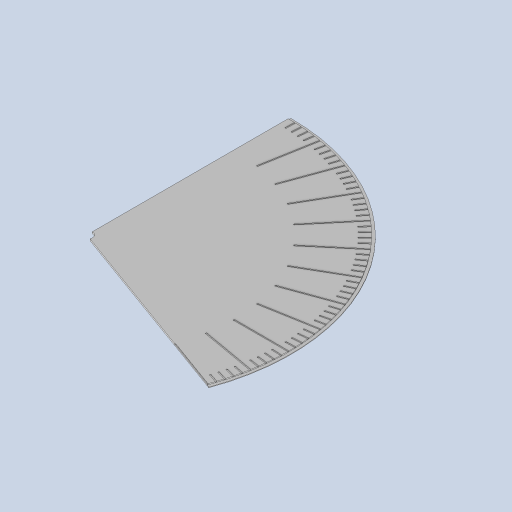
# Autodesk Inventor part: back_angler
Saved by Autodesk Inventor 2024.1 (Build 281209000, 209)
## iProperties
Created: 2023-12-04
Part Number: back_angler
Material: Generic
Document SubType Name: Modeling
Designer: dsdan
Density: 1 g/cm^3
Appearance: Default
Author: dsdan
Autodesk Inventor part; units mm, degrees
ref_plane "YZ Plane" through (0, 0, 0) normal (1, 0, 0) x (0, 1, 0)
ref_plane "XZ Plane" through (0, 0, 0) normal (0, 1, 0) x (-1, 0, 0)
ref_plane "XY Plane" through (0, 0, 0) normal (0, 0, 1) x (1, 0, 0)
sketch "Sketch1" plane through (0, 0, 0) normal (0, 1, 0) x (-1, 0, 0)
  circle A0 centre (0, 0) radius 111.8
  line L0 (0, 111.8) -> (0, -111.8)
  dimension "d0" = 223.6
  constraints: 2 end point, 2 point on circle, 1 centre point, 1 coincident, 1 vertical
  measures "d0" diameter of A0
extrude "Extrusion1" add sketch "Sketch1" along normal blind 0.6 contours L0 A0 picked at (-22.6865, 29.5656)
sketch "Sketch2" plane through (0, 0.6, 0) normal (0, 1, 0) x (1, 0, 0)
  arc A0 (0, -111.8) -> (0, 111.8) centre (0, 0) ccw projected
  line L0 (0, 111.8) -> (0, -111.8) projected
  line L1 (3.9018, -111.7319) -> (3.7272, -106.7319)
  line L2 (19.7832, -110.0364) -> (14.5737, -80.4922)
  line L3 (13.8351, -80.6224) -> (19.0446, -110.1666)
  arc A1 (19.0446, -110.1666) -> (19.7832, -110.0364) centre (19.4139, -110.1015) ccw
  arc A2 (14.5737, -80.4922) -> (13.8351, -80.6224) centre (14.2044, -80.5573) ccw
  line L4 (3.7272, -106.7319) -> (3.9018, -111.7319) construction
  line L5 (3.3524, -106.745) -> (3.527, -111.745)
  line L6 (4.2765, -111.7188) -> (4.1019, -106.7188)
  arc A3 (4.1019, -106.7188) -> (3.3524, -106.745) centre (3.7272, -106.7319) ccw
  arc A4 (3.527, -111.745) -> (4.2765, -111.7188) centre (3.9018, -111.7319) ccw
  line L7 (19.4139, -110.1015) -> (14.2044, -80.5573)
  point P0 (3.8145, -109.2319)
  point P1 (3.527, -111.7444)
  point P2 (4.2765, -111.7182)
  dimension "d9" = 5
  dimension "d14" = 0.75
  dimension "d15" = 0.75
  dimension "d26" = 2
  dimension "d27" = 30
  dimension "d28" = 10
  constraints: 16 end point, 10 point on circle, 8 tangent, 4 centre point, 3 midpoint, 2 parallel, 2 point on line
  measures "d9" vertical distance of L1.start L1.end
  measures "d14" diameter of A2
  measures "d15" diameter of A4
  measures "d26" angle of L0 L1
  measures "d27" distance of L7.start L7.end
  measures "d28" angle of L0 L7
extrude "Extrusion2" cut sketch "Sketch2" against normal blind 0.3 contours A0 A4 | A1 A0 | A0 L3 A2 L2
extrude "Extrusion3" cut sketch "Sketch2" against normal blind 0.3 contours L5 A3 L6 A0
pattern_circular "Circular Pattern1" count 89 over 176 about axis through (0, -10, 0) along (0, 1, 0) of "Extrusion3"
pattern_circular "Circular Pattern2" count 17 over 160 about axis through (0, -10, 0) along (0, 1, 0) of "Extrusion2"
sketch "Sketch3" plane through (0, 0.6, 0) normal (0, 1, 0) x (1, 0, 0)
  circle A0 centre (0, 0) radius 3
  dimension "d29" = 6
  constraints: 1 centre point, 1 coincident
  measures "d29" diameter of A0
extrude "Extrusion4" cut sketch "Sketch3" against normal through all
sketch "Sketch4" plane through (0, 0, 0) normal (0, -1, 0) x (1, 0, 0)
  arc A0 (0, -3) -> (0, 3) centre (0, 0) ccw projected
  line L0 (0, -111.8) -> (0, -3) projected
  arc A1 (0, -111.8) -> (0, 111.8) centre (0, 0) ccw projected
  line L1 (0, 3) -> (0, 111.8) projected
  arc A2 (-1.5, -113.2901) -> (-1.5, 113.2901) centre (0, 0) ccw
  line L2 (0, -111.8) -> (0, -113.3)
  line L3 (0, 111.8) -> (0, 113.3)
  dimension "d32" = 1.5
  constraints: 4 end point, 4 point on circle, 1 centre point, 1 point on line, 1 vertical
  measures "d32" radial gap between concentric circles of A1 A2
extrude "Extrusion5" add sketch "Sketch4" along normal blind 0.3
sketch "Sketch5" plane through (0, 0.6, 0) normal (0, 1, 0) x (1, 0, 0)
  arc A0 (0, -3) -> (0, 3) centre (0, 0) ccw projected
  line L0 (0, 0) -> (106.4672, -38.7509)
  arc A1 (0, -113.3) -> (0, 113.3) centre (0, 0) ccw projected
  line L1 (76.9951, -27.6249) -> (105.1853, -37.8853) projected
  constraints: 2 end point, 1 parallel, 1 point on circle
split body "Split1" sketch "Sketch5" result two bodies curves L0 first body at (67.6922, 0.2, -35.3628)
body "Solid2"
body "Solid3"
